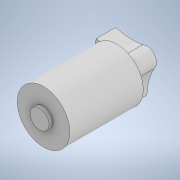
# Autodesk Inventor part: Vibration_motor
Saved by Autodesk Inventor 2021.4 (Build 254397000, 397)
## iProperties
Created: 2024-09-20
Part Number: Vibration_motor
Material: 一般
Document SubType Name: Modeling
Designer: hikou
Density: 1 g/cm^3
Appearance: 既定
Author: hikou
Autodesk Inventor part; units mm, degrees
ref_plane "YZ Plane" through (0, 0, 0) normal (1, 0, 0) x (0, 1, 0)
ref_plane "XZ Plane" through (0, 0, 0) normal (0, 1, 0) x (-1, 0, 0)
ref_plane "XY Plane" through (0, 0, 0) normal (0, 0, 1) x (1, 0, 0)
sketch "スケッチ1" plane through (0, 0, 0) normal (0, 0, 1) x (1, 0, 0)
  circle A0 centre (0, 0) radius 13.6
  dimension "d0" = 27.2
  constraints: 1 centre point, 1 coincident
  measures "d0" diameter of A0
extrude "押し出し1" add sketch "スケッチ1" along normal mid plane 38
sketch "スケッチ2" plane through (0, 0, 19) normal (0, 0, 1) x (1, 0, 0)
  circle A0 centre (0, 0) radius 4.9
  dimension "d3" = 9.8
  constraints: 1 centre point, 1 coincident
  measures "d3" diameter of A0
extrude "押し出し2" add sketch "スケッチ2" along normal blind 2
sketch "スケッチ3" plane through (0, 0, -19) normal (0, 0, -1) x (-1, 0, 0)
  circle A0 centre (0, 0) radius 4.85
  dimension "d6" = 9.7
  constraints: 1 centre point, 1 coincident
  measures "d6" diameter of A0
extrude "押し出し3" add sketch "スケッチ3" along normal blind 2.5
sketch "スケッチ4" plane through (0, 0, -21.5) normal (0, 0, -1) x (-1, 0, 0)
  circle A0 centre (0, 0) radius 4.85 projected
  circle A1 centre (0, 0) radius 1
  dimension "d9" = 2
  constraints: 1 centre point, 1 coincident
  measures "d9" diameter of A1
extrude "押し出し4" add sketch "スケッチ4" along normal blind 3 contours A1
sketch "スケッチ5" plane through (0, 0, -24.5) normal (0, 0, -1) x (-1, 0, 0)
  circle A0 centre (0, 0) radius 5
  circle A1 centre (0, 0) radius 1 projected
  circle A2 centre (0, 0) radius 17
  line L0 (0, 0) -> (0, -17)
  line L1 (0, 0) -> (16.168, 5.2533)
  circle A3 centre (0, 0) radius 4.85 projected
  line L2 (0, 0) -> (-4.7553, -1.5451)
  line L3 (0, 0) -> (0, 5)
  arc A4 (0, -17) -> (-4.7553, -1.5451) centre (-29.9902, -17.7686) ccw
  arc A5 (0, 5) -> (16.168, 5.2533) centre (7.6314, 34.0131) ccw
  point P0 (2.1361, 4.5207)
  point P1 (-3.6394, -3.4286)
  dimension "d12" = 10
  dimension "d13" = 34
  dimension "d14" = 108
  dimension "d15" = 108
  dimension "d16" = 72
  dimension "d17" = 30
  dimension "d18" = 30
  constraints: 10 point on circle, 8 end point, 4 centre point, 2 coincident, 1 vertical
  measures "d12" diameter of A0
  measures "d13" diameter of A2
  measures "d14" angle of L0 L1
  measures "d15" angle of L3 L2
  measures "d16" angle of L0 L2
  measures "d17" radius of A4
  measures "d18" radius of A5
extrude "押し出し5" add sketch "スケッチ5" along normal blind 10 contours L3 A3 L2 A0 | A5 A0 L1 A3 L3 | A0 A5 | A4 A0 | L2 A3 L0 A0 A4 | A5 L1 A0 | L3 A1 L2 A3 | A3 L1 A1 L3 | A0 L0 A4 | L2 A1 L0 A3 | L1 A2 L0 A0 | A0 L0 A3 L1 | A3 L0 A1 L1 | L3 L2 A1 | A1 L1 L3 | L2 L0 A1 | A1 L0 L1
sketch "スケッチ6" plane through (0, 0, -19) normal (0, 0, -1) x (-1, 0, 0)
  circle A0 centre (0, 0) radius 4.85 projected
  circle A1 centre (0, 0) radius 13.6 projected
  point P0 (0, 8.6)
  point P1 (0, -8.6)
  dimension "d21" = 8.6
  dimension "d22" = 8.6
  measures "d21" distance of A1.centre point (0, 8.6)
  measures "d22" distance of A1.centre point (0, -8.6)
hole "穴1" at (0, 8.6, -19) at (0, -8.6, -19) direction (0, 0, 1) diameter 1.7294 depth 5.5 tip angle 118 thread size "M2x0.25" class "6H" standard "ISO Metric profile"
equation "\"d15\" = d14"
equation "\"d22\" = d21"
